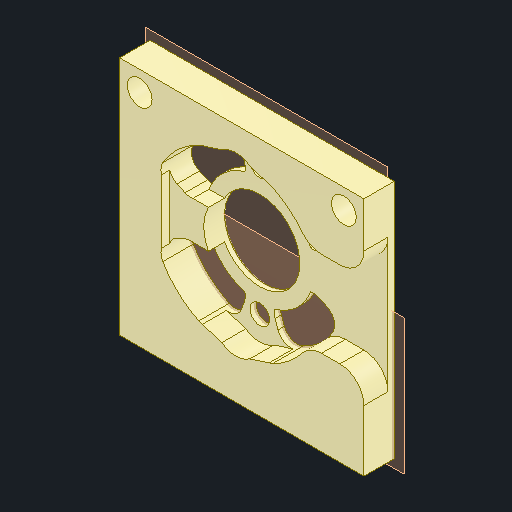
# Autodesk Inventor part: front_motur_holder
Saved by Autodesk Inventor 2023 (Build 270158000, 158)
## iProperties
Created: 2024-04-30
Part Number: front_motur_holder
Material: Nylon 6/6
Document SubType Name: Modeling
Designer: szymo
Density: 1.13 g/cm^3
Appearance: Nylon 6
Mass: 2.32105 g
Surface Area: 21.928 cm^2
Volume: 2.05403 cm^3
Author: szymo
Autodesk Inventor part; units mm, degrees
ref_plane "YZ Plane" through (0, 0, 0) normal (1, 0, 0) x (0, 1, 0)
ref_plane "XZ Plane" through (0, 0, 0) normal (0, 1, 0) x (-1, 0, 0)
ref_plane "XY Plane" through (0, 0, 0) normal (0, 0, 1) x (1, 0, 0)
ref_plane "Work Plane1" through (0, 0, 0) normal (0, 0, 1) x (1, 0, 0)
ref_plane "Work Plane2" through (-0.625, 8.3125, -0.3) normal (0, 0, 1) x (0, 1, 0)
sketch "Sketch6" plane through (-0.625, 8.3125, -0.3) normal (0, 0, 1) x (0, 1, 0)
  line L0 (-3.58, 8.0542) -> (-3.1299, 7.0416) projected
  arc A0 (-3.5233, 5.7815) -> (-3.1299, 7.0416) centre (-4.0437, 6.6354) ccw projected
  arc A1 (-3.5233, 5.7815) -> (-6.0426, 3.0539) centre (0, 0) ccw projected
  arc A2 (-7.2676, 2.5618) -> (-6.0426, 3.0539) centre (-6.9351, 3.5049) ccw projected
  line L1 (-7.2676, 2.5618) -> (-8.3126, 2.9302) projected
  arc A3 (-8.8798, 4.3099) -> (-8.3126, 2.9302) centre (-7.9802, 3.8733) ccw projected
  arc A4 (-5.0004, 8.5102) -> (-8.8798, 4.3099) centre (0, 0) ccw projected
  arc A5 (-3.58, 8.0542) -> (-5.0004, 8.5102) centre (-4.4938, 7.648) ccw projected
  line L2 (-3.1299, -7.0416) -> (-3.58, -8.0542) projected
  arc A6 (-5.0004, -8.5102) -> (-3.58, -8.0542) centre (-4.4938, -7.648) ccw projected
  arc A7 (-8.8798, -4.3099) -> (-5.0004, -8.5102) centre (0, 0) ccw projected
  arc A8 (-8.3126, -2.9302) -> (-8.8798, -4.3099) centre (-7.9802, -3.8733) ccw projected
  line L3 (-8.3126, -2.9302) -> (-7.2676, -2.5618) projected
  arc A9 (-6.0426, -3.0539) -> (-7.2676, -2.5618) centre (-6.9351, -3.5049) ccw projected
  arc A10 (-6.0426, -3.0539) -> (-3.5233, -5.7815) centre (0, 0) ccw projected
  arc A11 (-3.1299, -7.0416) -> (-3.5233, -5.7815) centre (-4.0437, -6.6354) ccw projected
  line L4 (3.1299, 7.0416) -> (3.58, 8.0542) projected
  arc A12 (5.0004, 8.5102) -> (3.58, 8.0542) centre (4.4938, 7.648) ccw projected
  arc A13 (8.8798, 4.3099) -> (5.0004, 8.5102) centre (0, 0) ccw projected
  arc A14 (8.3126, 2.9302) -> (8.8798, 4.3099) centre (7.9802, 3.8733) ccw projected
  line L5 (8.3126, 2.9302) -> (7.2676, 2.5618) projected
  arc A15 (6.0426, 3.0539) -> (7.2676, 2.5618) centre (6.9351, 3.5049) ccw projected
  arc A16 (6.0426, 3.0539) -> (3.5233, 5.7815) centre (0, 0) ccw projected
  arc A17 (3.1299, 7.0416) -> (3.5233, 5.7815) centre (4.0437, 6.6354) ccw projected
  line L6 (3.58, -8.0542) -> (3.1299, -7.0416) projected
  arc A18 (3.5233, -5.7815) -> (3.1299, -7.0416) centre (4.0437, -6.6354) ccw projected
  arc A19 (3.5233, -5.7815) -> (6.0426, -3.0539) centre (0, 0) ccw projected
  arc A20 (7.2676, -2.5618) -> (6.0426, -3.0539) centre (6.9351, -3.5049) ccw projected
  line L7 (7.2676, -2.5618) -> (8.3126, -2.9302) projected
  arc A21 (8.8798, -4.3099) -> (8.3126, -2.9302) centre (7.9802, -3.8733) ccw projected
  arc A22 (5.0004, -8.5102) -> (8.8798, -4.3099) centre (0, 0) ccw projected
  arc A23 (3.58, -8.0542) -> (5.0004, -8.5102) centre (4.4938, -7.648) ccw projected
  circle A24 centre (8, 0) radius 1.2295 projected
  circle A25 centre (-8, 0) radius 1.2295 projected
  circle A26 centre (0, 0) radius 5 projected
  circle A27 centre (0, 0) radius 13.75 projected
  line L8 (-10, 15.75) -> (14, 15.75) projected
  line L9 (-10, 15.75) -> (-10, 9.4373) projected
  arc A28 (-10, 9.4373) -> (-0.3764, -13.7448) centre (0, 0) ccw projected
  line L10 (-0.3764, -13.7448) -> (-1, -16) projected
  line L11 (14, -16) -> (-1, -16) projected
  line L12 (14, 15.75) -> (14, -16) projected
  line L13 (14, -16) -> (-16, -16)
  line L14 (-16, -16) -> (-16, 14.5)
  line L15 (-16, 14.5) -> (14, 14.5)
  line L16 (14, 14.5) -> (14, -16)
  line L17 (-19.5, 96) -> (-19.5, -16) projected
  line L18 (-19.5, -16) -> (-16, -16) projected
  line L19 (-16, 96) -> (-16, -16) projected
  line L20 (-19.5, 96) -> (-16, 96) projected
  arc A29 (3.1299, 7.0416) -> (3.5233, 5.7815) centre (4.0437, 6.6354) ccw projected
  arc A30 (6.0426, 3.0539) -> (3.5233, 5.7815) centre (0, 0) ccw projected
  arc A31 (6.0426, 3.0539) -> (7.2676, 2.5618) centre (6.9351, 3.5049) ccw projected
  line L21 (8.3126, 2.9302) -> (7.2676, 2.5618) projected
  arc A32 (8.3126, 2.9302) -> (8.8798, 4.3099) centre (7.9802, 3.8733) ccw projected
  arc A33 (8.8798, 4.3099) -> (5.0004, 8.5102) centre (0, 0) ccw projected
  arc A34 (5.0004, 8.5102) -> (3.58, 8.0542) centre (4.4938, 7.648) ccw projected
  line L22 (3.1299, 7.0416) -> (3.58, 8.0542) projected
  arc A35 (8.8798, -4.3099) -> (8.3126, -2.9302) centre (7.9802, -3.8733) ccw projected
  line L23 (7.2676, -2.5618) -> (8.3126, -2.9302) projected
  arc A36 (7.2676, -2.5618) -> (6.0426, -3.0539) centre (6.9351, -3.5049) ccw projected
  arc A37 (3.5233, -5.7815) -> (6.0426, -3.0539) centre (0, 0) ccw projected
  arc A38 (3.5233, -5.7815) -> (3.1299, -7.0416) centre (4.0437, -6.6354) ccw projected
  line L24 (3.58, -8.0542) -> (3.1299, -7.0416) projected
  arc A39 (3.58, -8.0542) -> (5.0004, -8.5102) centre (4.4938, -7.648) ccw projected
  arc A40 (5.0004, -8.5102) -> (8.8798, -4.3099) centre (0, 0) ccw projected
  arc A41 (-3.1299, -7.0416) -> (-3.5233, -5.7815) centre (-4.0437, -6.6354) ccw projected
  arc A42 (-6.0426, -3.0539) -> (-3.5233, -5.7815) centre (0, 0) ccw projected
  arc A43 (-6.0426, -3.0539) -> (-7.2676, -2.5618) centre (-6.9351, -3.5049) ccw projected
  line L25 (-8.3126, -2.9302) -> (-7.2676, -2.5618) projected
  arc A44 (-8.3126, -2.9302) -> (-8.8798, -4.3099) centre (-7.9802, -3.8733) ccw projected
  arc A45 (-8.8798, -4.3099) -> (-5.0004, -8.5102) centre (0, 0) ccw projected
  arc A46 (-5.0004, -8.5102) -> (-3.58, -8.0542) centre (-4.4938, -7.648) ccw projected
  line L26 (-3.1299, -7.0416) -> (-3.58, -8.0542) projected
  arc A47 (-3.5233, 5.7815) -> (-3.1299, 7.0416) centre (-4.0437, 6.6354) ccw projected
  line L27 (-3.58, 8.0542) -> (-3.1299, 7.0416) projected
  arc A48 (-3.58, 8.0542) -> (-5.0004, 8.5102) centre (-4.4938, 7.648) ccw projected
  arc A49 (-5.0004, 8.5102) -> (-8.8798, 4.3099) centre (0, 0) ccw projected
  arc A50 (-8.8798, 4.3099) -> (-8.3126, 2.9302) centre (-7.9802, 3.8733) ccw projected
  line L28 (-7.2676, 2.5618) -> (-8.3126, 2.9302) projected
  arc A51 (-7.2676, 2.5618) -> (-6.0426, 3.0539) centre (-6.9351, 3.5049) ccw projected
  arc A52 (-3.5233, 5.7815) -> (-6.0426, 3.0539) centre (0, 0) ccw projected
  circle A53 centre (0, 0) radius 6.7705
  arc A54 (2.4903, 7.3259) -> (2.3692, 6.3425) centre (4.0437, 6.6354) ccw
  line L29 (2.4903, 7.3259) -> (2.9403, 8.3385)
  arc A55 (5.355, 9.1137) -> (2.9403, 8.3385) centre (4.4938, 7.648) ccw
  arc A56 (9.5096, 4.6156) -> (5.355, 9.1137) centre (0, 0) ccw
  arc A57 (8.5453, 2.27) -> (9.5096, 4.6156) centre (7.9802, 3.8733) ccw
  line L30 (8.5453, 2.27) -> (7.5003, 1.9016)
  arc A58 (6.5103, 1.8588) -> (7.5003, 1.9016) centre (6.9351, 3.5049) ccw
  arc A59 (7.5003, -1.9016) -> (6.5103, -1.8588) centre (6.9351, -3.5049) ccw
  line L31 (7.5003, -1.9016) -> (8.5453, -2.27)
  arc A60 (9.5096, -4.6156) -> (8.5453, -2.27) centre (7.9802, -3.8733) ccw
  arc A61 (5.355, -9.1137) -> (9.5096, -4.6156) centre (0, 0) ccw
  arc A62 (2.9403, -8.3385) -> (5.355, -9.1137) centre (4.4938, -7.648) ccw
  line L32 (2.9403, -8.3385) -> (2.4903, -7.3259)
  arc A63 (2.3692, -6.3425) -> (2.4903, -7.3259) centre (4.0437, -6.6354) ccw
  arc A64 (-2.4903, -7.3259) -> (-2.3692, -6.3425) centre (-4.0437, -6.6354) ccw
  line L33 (-2.4903, -7.3259) -> (-2.9403, -8.3385)
  arc A65 (-5.355, -9.1137) -> (-2.9403, -8.3385) centre (-4.4938, -7.648) ccw
  arc A66 (-9.5096, -4.6156) -> (-5.355, -9.1137) centre (0, 0) ccw
  arc A67 (-8.5453, -2.27) -> (-9.5096, -4.6156) centre (-7.9802, -3.8733) ccw
  line L34 (-8.5453, -2.27) -> (-7.5003, -1.9016)
  arc A68 (-6.5103, -1.8588) -> (-7.5003, -1.9016) centre (-6.9351, -3.5049) ccw
  arc A69 (-7.5003, 1.9016) -> (-6.5103, 1.8588) centre (-6.9351, 3.5049) ccw
  line L35 (-7.5003, 1.9016) -> (-8.5453, 2.27)
  arc A70 (-9.5096, 4.6156) -> (-8.5453, 2.27) centre (-7.9802, 3.8733) ccw
  arc A71 (-5.355, 9.1137) -> (-9.5096, 4.6156) centre (0, 0) ccw
  arc A72 (-2.9403, 8.3385) -> (-5.355, 9.1137) centre (-4.4938, 7.648) ccw
  line L36 (-2.9403, 8.3385) -> (-2.4903, 7.3259)
  arc A73 (-2.3692, 6.3425) -> (-2.4903, 7.3259) centre (-4.0437, 6.6354) ccw
  point P0 (-8.3125, -0.625)
  point P1 (2.4903, 7.3259)
  point P2 (2.9403, 8.3385)
  point P3 (9.5096, 4.6156)
  point P4 (8.5453, 2.27)
  point P5 (7.5003, 1.9016)
  point P6 (3.5233, 5.7815)
  point P7 (-3.5233, 5.7815)
  point P8 (-6.0426, 3.0539)
  point P9 (-8.5453, 2.27)
  point P10 (-5.355, 9.1137)
  point P11 (-2.4903, 7.3259)
  point P12 (-3.5233, -5.7815)
  point P13 (-2.4903, -7.3259)
  point P14 (-2.9403, -8.3385)
  point P15 (-8.5453, -2.27)
  point P16 (3.5233, -5.7815)
  point P17 (6.0426, -3.0539)
  point P18 (7.5003, -1.9016)
  point P19 (8.5453, -2.27)
  point P20 (9.5096, -4.6156)
  point P21 (5.355, -9.1137)
  point P22 (2.9403, -8.3385)
  point P23 (2.4903, -7.3259)
  point P24 (14, 14.5)
  dimension "d39" = 16
  dimension "d40" = 14.5
  dimension "d41" = 0.7
  dimension "d42" = 0.7
  dimension "d43" = 0.7
  dimension "d44" = 0.7
  dimension "d45" = 0.7
  dimension "d46" = 0.7
  dimension "d47" = 0.7
  dimension "d48" = 0.7
  dimension "d49" = 0.7
  dimension "d50" = 0.7
  dimension "d51" = 0.7
  dimension "d52" = 0.7
  dimension "d53" = 0.7
  dimension "d54" = 0.7
  dimension "d55" = 0.7
  dimension "d56" = 0.7
  dimension "d57" = 0.7
  dimension "d58" = 0.7
  dimension "d59" = 0.7
  dimension "d60" = 0.7
  dimension "d61" = 0.7
  dimension "d62" = 0.7
  dimension "d63" = 0.7
  dimension "d64" = 0.7
  dimension "d65" = 0.7
  dimension "d66" = 0.7
  dimension "d67" = 0.7
  dimension "d68" = 0.7
  constraints: 40 point on circle, 24 end point, 20 centre point, 10 parallel, 1 coincident, 1 horizontal, 1 perpendicular, 1 point on line, 11 other
  measures "d39" distance from line of L11 A1.centre
  measures "d40" distance from line of L15 A1.centre
  measures "d41" radial gap between concentric circles of A17 A54
  measures "d42" distance between parallel lines of L4 L29
  measures "d43" radial gap between concentric circles of A12 A55
  measures "d44" radial gap between concentric circles of A13 A56
  measures "d45" radial gap between concentric circles of A14 A57
  measures "d46" distance between parallel lines of L5 L30
  measures "d47" radial gap between concentric circles of A15 A58
  measures "d48" radial gap between concentric circles of A20 A59
  measures "d49" distance between parallel lines of L7 L31
  measures "d50" radial gap between concentric circles of A35 A60
  measures "d51" radial gap between concentric circles of A40 A61
  measures "d52" radial gap between concentric circles of A39 A62
  measures "d53" distance between parallel lines of L6 L32
  measures "d54" radial gap between concentric circles of A18 A63
  measures "d55" radial gap between concentric circles of A11 A64
  measures "d56" distance between parallel lines of L26 L33
  measures "d57" radial gap between concentric circles of A6 A65
  measures "d58" radial gap between concentric circles of A45 A66
  measures "d59" radial gap between concentric circles of A44 A67
  measures "d60" distance between parallel lines of L3 L34
  measures "d61" radial gap between concentric circles of A9 A68
  measures "d62" radial gap between concentric circles of A2 A69
  measures "d63" distance between parallel lines of L28 L35
  measures "d64" radial gap between concentric circles of A3 A70
  measures "d65" radial gap between concentric circles of A4 A71
  measures "d66" radial gap between concentric circles of A5 A72
  measures "d67" distance between parallel lines of L27 L36
  measures "d68" radial gap between concentric circles of A47 A73
extrude "Extrusion4" add sketch "Sketch6" along normal blind 0.8 contours A53 A16 A19 A10 A1 | A27 | A27 L9 L15 L12 L11 L10 | A27 L10 L13 L14 L15 L9
sketch "Sketch7" plane through (-0.625, 8.3125, 0.5) normal (0, 0, 1) x (1, 0, 0)
  arc A0 (-7.3259, 2.4903) -> (-6.3425, 2.3692) centre (-6.6354, 4.0437) ccw projected
  line L0 (-7.3259, 2.4903) -> (-8.3385, 2.9403) projected
  arc A1 (-9.1137, 5.355) -> (-8.3385, 2.9403) centre (-7.648, 4.4938) ccw projected
  arc A2 (-4.6156, 9.5096) -> (-9.1137, 5.355) centre (0, 0) ccw projected
  arc A3 (-2.27, 8.5453) -> (-4.6156, 9.5096) centre (-3.8733, 7.9802) ccw projected
  line L1 (-2.27, 8.5453) -> (-1.9016, 7.5003) projected
  arc A4 (-1.8588, 6.5103) -> (-1.9016, 7.5003) centre (-3.5049, 6.9351) ccw projected
  arc A5 (-1.8588, 6.5103) -> (-6.3425, 2.3692) centre (0, 0) ccw projected
  arc A6 (-6.3425, -2.3692) -> (-1.8588, -6.5103) centre (0, 0) ccw projected
  arc A7 (-1.9016, -7.5003) -> (-1.8588, -6.5103) centre (-3.5049, -6.9351) ccw projected
  line L2 (-1.9016, -7.5003) -> (-2.27, -8.5453) projected
  arc A8 (-4.6156, -9.5096) -> (-2.27, -8.5453) centre (-3.8733, -7.9802) ccw projected
  arc A9 (-9.1137, -5.355) -> (-4.6156, -9.5096) centre (0, 0) ccw projected
  arc A10 (-8.3385, -2.9403) -> (-9.1137, -5.355) centre (-7.648, -4.4938) ccw projected
  line L3 (-8.3385, -2.9403) -> (-7.3259, -2.4903) projected
  arc A11 (-6.3425, -2.3692) -> (-7.3259, -2.4903) centre (-6.6354, -4.0437) ccw projected
  circle A12 centre (0, -8) radius 1.2295 projected
  arc A13 (1.8588, -6.5103) -> (6.3425, -2.3692) centre (0, 0) ccw projected
  arc A14 (7.3259, -2.4903) -> (6.3425, -2.3692) centre (6.6354, -4.0437) ccw projected
  line L4 (7.3259, -2.4903) -> (8.3385, -2.9403) projected
  arc A15 (9.1137, -5.355) -> (8.3385, -2.9403) centre (7.648, -4.4938) ccw projected
  arc A16 (4.6156, -9.5096) -> (9.1137, -5.355) centre (0, 0) ccw projected
  arc A17 (2.27, -8.5453) -> (4.6156, -9.5096) centre (3.8733, -7.9802) ccw projected
  line L5 (2.27, -8.5453) -> (1.9016, -7.5003) projected
  arc A18 (1.8588, -6.5103) -> (1.9016, -7.5003) centre (3.5049, -6.9351) ccw projected
  arc A19 (6.3425, 2.3692) -> (1.8588, 6.5103) centre (0, 0) ccw projected
  arc A20 (1.9016, 7.5003) -> (1.8588, 6.5103) centre (3.5049, 6.9351) ccw projected
  line L6 (1.9016, 7.5003) -> (2.27, 8.5453) projected
  arc A21 (4.6156, 9.5096) -> (2.27, 8.5453) centre (3.8733, 7.9802) ccw projected
  arc A22 (9.1137, 5.355) -> (4.6156, 9.5096) centre (0, 0) ccw projected
  arc A23 (8.3385, 2.9403) -> (9.1137, 5.355) centre (7.648, 4.4938) ccw projected
  line L7 (8.3385, 2.9403) -> (7.3259, 2.4903) projected
  arc A24 (6.3425, 2.3692) -> (7.3259, 2.4903) centre (6.6354, 4.0437) ccw projected
  circle A25 centre (0, 0) radius 5 projected
  circle A26 centre (0, 8) radius 1.2295 projected
  line L8 (-14.5, 14) -> (-14.5, -16) projected
  line L9 (-14.5, -16) -> (16, -16) projected
  line L10 (16, -16) -> (16, 14) projected
  line L11 (16, 14) -> (-14.5, 14) projected
  circle A27 centre (0, 8) radius 3
  circle A28 centre (0, -8) radius 1.2295 projected
  circle A29 centre (0, -8) radius 3
  arc A30 (9.1137, 5.355) -> (4.6156, 9.5096) centre (0, 0) ccw projected
  line L12 (9.1137, 5.355) -> (16, 5.355)
  line L13 (16, -16) -> (16, 14) projected
  arc A31 (9.1137, -5.355) -> (8.3385, -2.9403) centre (7.648, -4.4938) ccw projected
  line L14 (9.1137, -5.355) -> (16, -5.355)
  arc A32 (4.6156, 9.5096) -> (2.27, 8.5453) centre (3.8733, 7.9802) ccw projected
  line L15 (4.6156, 9.5096) -> (0, 11)
  arc A33 (-2.27, 8.5453) -> (-4.6156, 9.5096) centre (-3.8733, 7.9802) ccw projected
  line L16 (-4.6156, 9.5096) -> (0, 11)
  arc A34 (-9.1137, 5.355) -> (-8.3385, 2.9403) centre (-7.648, 4.4938) ccw projected
  line L17 (-9.2666, 3.9741) -> (-9.2666, -3.9741)
  arc A35 (-8.3385, -2.9403) -> (-9.1137, -5.355) centre (-7.648, -4.4938) ccw projected
  arc A36 (-4.6156, -9.5096) -> (-2.27, -8.5453) centre (-3.8733, -7.9802) ccw projected
  line L18 (-4.6156, -9.5096) -> (0, -11)
  arc A37 (2.27, -8.5453) -> (4.6156, -9.5096) centre (3.8733, -7.9802) ccw projected
  line L19 (0, -11) -> (4.6156, -9.5096)
  line L20 (-6.3425, 2.3692) -> (-4.4031, 2.3692)
  circle A38 centre (0, 0) radius 5 projected
  arc A39 (-6.3425, -2.3692) -> (-1.8588, -6.5103) centre (0, 0) ccw projected
  line L21 (-6.3425, -2.3692) -> (-4.4031, -2.3692)
  point P0 (0.625, -8.3125)
  point P1 (-4.1656, 9.6549)
  point P2 (-1.7545, 10.4334)
  point P3 (1.7545, 10.4334)
  point P4 (4.1656, 9.6549)
  point P5 (4.1656, -9.6549)
  point P6 (1.7545, -10.4334)
  point P7 (-1.7545, -10.4334)
  point P8 (-4.1656, -9.6549)
  point P9 (-2.4735, -6.3025)
  point P10 (0, -5)
  point P11 (0, 5)
  point P12 (-2.4735, 6.3025)
  dimension "d71" = 6
  dimension "d72" = 6
  constraints: 18 end point, 5 point on circle, 2 coincident, 2 horizontal, 2 parallel, 2 point on line, 10 other
extrude "Extrusion5" add sketch "Sketch7" along normal blind 2 contours A0 L20 A25 L21 A11 L3 A10 L17 A1 L0 | L17 A10 A9 A8 L18 A29 L19 A17 A16 L14 L10 L9 L8 L11 L12 A22 A21 L15 A27 L16 A3 A2 A1
fillet "Fillet1" radius 3 4 edges at (15.375, 13.6675, 1.5) (15.375, 2.9575, 1.5) (8.4887, 2.9575, 1.5) (8.4887, 13.6675, 1.5)
fillet "Fillet2" radius 0.2 1 edges at (-0.625, 3.3125, -0.3)
sketch "Sketch8" plane through (-0.625, 8.3125, -0.3) normal (0, 0, -1) x (-1, 0, 0)
  line L0 (14.5, 14) -> (14.5, -16) projected
  line L1 (-16, 14) -> (14.5, 14) projected
  line L2 (-16, -16) -> (-16, 14) projected
  line L3 (14.5, -16) -> (-16, -16) projected
  circle A0 centre (0, 8) radius 1.2295 projected
  arc A1 (-1.8588, 6.5103) -> (-6.3425, 2.3692) centre (0, 0) ccw projected
  arc A2 (-7.3259, 2.4903) -> (-6.3425, 2.3692) centre (-6.6354, 4.0437) ccw projected
  line L4 (-8.3385, 2.9403) -> (-7.3259, 2.4903) projected
  arc A3 (-9.1137, 5.355) -> (-8.3385, 2.9403) centre (-7.648, 4.4938) ccw projected
  arc A4 (-4.6156, 9.5096) -> (-9.1137, 5.355) centre (0, 0) ccw projected
  arc A5 (-2.27, 8.5453) -> (-4.6156, 9.5096) centre (-3.8733, 7.9802) ccw projected
  line L5 (-1.9016, 7.5003) -> (-2.27, 8.5453) projected
  arc A6 (-1.8588, 6.5103) -> (-1.9016, 7.5003) centre (-3.5049, 6.9351) ccw projected
  arc A7 (-6.3425, -2.3692) -> (-1.8588, -6.5103) centre (0, 0) ccw projected
  arc A8 (-1.9016, -7.5003) -> (-1.8588, -6.5103) centre (-3.5049, -6.9351) ccw projected
  line L6 (-2.27, -8.5453) -> (-1.9016, -7.5003) projected
  arc A9 (-4.6156, -9.5096) -> (-2.27, -8.5453) centre (-3.8733, -7.9802) ccw projected
  arc A10 (-9.1137, -5.355) -> (-4.6156, -9.5096) centre (0, 0) ccw projected
  arc A11 (-8.3385, -2.9403) -> (-9.1137, -5.355) centre (-7.648, -4.4938) ccw projected
  line L7 (-7.3259, -2.4903) -> (-8.3385, -2.9403) projected
  arc A12 (-6.3425, -2.3692) -> (-7.3259, -2.4903) centre (-6.6354, -4.0437) ccw projected
  circle A13 centre (0, -8) radius 1.2295 projected
  arc A14 (1.8588, -6.5103) -> (6.3425, -2.3692) centre (0, 0) ccw projected
  arc A15 (7.3259, -2.4903) -> (6.3425, -2.3692) centre (6.6354, -4.0437) ccw projected
  line L8 (8.3385, -2.9403) -> (7.3259, -2.4903) projected
  arc A16 (9.1137, -5.355) -> (8.3385, -2.9403) centre (7.648, -4.4938) ccw projected
  arc A17 (4.6156, -9.5096) -> (9.1137, -5.355) centre (0, 0) ccw projected
  arc A18 (2.27, -8.5453) -> (4.6156, -9.5096) centre (3.8733, -7.9802) ccw projected
  line L9 (1.9016, -7.5003) -> (2.27, -8.5453) projected
  arc A19 (1.8588, -6.5103) -> (1.9016, -7.5003) centre (3.5049, -6.9351) ccw projected
  arc A20 (6.3425, 2.3692) -> (7.3259, 2.4903) centre (6.6354, 4.0437) ccw projected
  arc A21 (6.3425, 2.3692) -> (1.8588, 6.5103) centre (0, 0) ccw projected
  arc A22 (1.9016, 7.5003) -> (1.8588, 6.5103) centre (3.5049, 6.9351) ccw projected
  line L10 (2.27, 8.5453) -> (1.9016, 7.5003) projected
  arc A23 (4.6156, 9.5096) -> (2.27, 8.5453) centre (3.8733, 7.9802) ccw projected
  arc A24 (9.1137, 5.355) -> (4.6156, 9.5096) centre (0, 0) ccw projected
  arc A25 (8.3385, 2.9403) -> (9.1137, 5.355) centre (7.648, 4.4938) ccw projected
  line L11 (7.3259, 2.4903) -> (8.3385, 2.9403) projected
  circle A26 centre (0, 0) radius 5.2 projected
  circle A27 centre (-13.5, 11.5) radius 2.5
  circle A28 centre (12, 11.5) radius 2.5
  point P0 (-0.625, -8.3125)
  dimension "d77" = 5
  dimension "d78" = 2.5
  dimension "d79" = 2.5
  dimension "d80" = 5
  dimension "d81" = 2.5
  dimension "d82" = 2.5
  constraints: 2 centre point, 2 coincident
  measures "d77" diameter of A27
  measures "d78" distance from line of L1 A27.centre
  measures "d79" distance from line of L2 A27.centre
  measures "d80" diameter of A28
  measures "d81" distance from line of L1 A28.centre
  measures "d82" distance from line of L0 A28.centre
hole "Hole3" at (12.875, 19.8125, -0.3) at (-12.625, 19.8125, -0.3) direction (0, 0, 1) diameter 3.1 end through all countersink diameter 5 countersink angle 90 clearance for "Countersunk Flat Head Screw ISO 2009/7046" size "M2.5" standard "ISO"
sketch "Sketch9" plane through (-0.625, 8.3125, 2.5) normal (0, 0, 1) x (1, 0, 0)
  circle A0 centre (13.5, 11.5) radius 1.55 projected
  circle A1 centre (-12, 11.5) radius 1.55 projected
  arc A2 (8.3296, 6.508) -> (10.6936, 5.355) centre (10.6936, 8.355) ccw projected
  line L0 (10.6936, 5.355) -> (13, 5.355) projected
  arc A3 (13, 5.355) -> (16, 8.355) centre (13, 8.355) ccw projected
  line L1 (16, 8.355) -> (16, 14) projected
  line L2 (16, 14) -> (-14.5, 14) projected
  line L3 (-14.5, 14) -> (-14.5, -16) projected
  line L4 (-14.5, -16) -> (16, -16) projected
  line L5 (16, -16) -> (16, -8.355) projected
  arc A4 (16, -8.355) -> (13, -5.355) centre (13, -8.355) ccw projected
  line L6 (13, -5.355) -> (10.6936, -5.355) projected
  arc A5 (10.6936, -5.355) -> (8.3296, -6.508) centre (10.6936, -8.355) ccw projected
  arc A6 (4.6156, -9.5096) -> (8.3296, -6.508) centre (0, 0) ccw projected
  arc A7 (4.1656, -9.6549) -> (4.6156, -9.5096) centre (3.8733, -7.9802) ccw projected
  line L7 (4.1656, -9.6549) -> (1.7545, -10.4334) projected
  arc A8 (-1.7545, -10.4334) -> (1.7545, -10.4334) centre (0, -8) ccw projected
  line L8 (-1.7545, -10.4334) -> (-4.1656, -9.6549) projected
  arc A9 (-4.6156, -9.5096) -> (-4.1656, -9.6549) centre (-3.8733, -7.9802) ccw projected
  arc A10 (-9.1137, -5.355) -> (-4.6156, -9.5096) centre (0, 0) ccw projected
  arc A11 (-8.3385, -2.9403) -> (-9.1137, -5.355) centre (-7.648, -4.4938) ccw projected
  line L9 (-8.3385, -2.9403) -> (-7.3259, -2.4903) projected
  arc A12 (-6.3425, -2.3692) -> (-7.3259, -2.4903) centre (-6.6354, -4.0437) ccw projected
  line L10 (-6.3425, -2.3692) -> (-4.4031, -2.3692) projected
  arc A13 (-4.4031, 2.3692) -> (-4.4031, -2.3692) centre (0, 0) ccw projected
  line L11 (-4.4031, 2.3692) -> (-6.3425, 2.3692) projected
  arc A14 (-7.3259, 2.4903) -> (-6.3425, 2.3692) centre (-6.6354, 4.0437) ccw projected
  line L12 (-7.3259, 2.4903) -> (-8.3385, 2.9403) projected
  arc A15 (-9.1137, 5.355) -> (-8.3385, 2.9403) centre (-7.648, 4.4938) ccw projected
  arc A16 (-4.6156, 9.5096) -> (-9.1137, 5.355) centre (0, 0) ccw projected
  arc A17 (-4.1656, 9.6549) -> (-4.6156, 9.5096) centre (-3.8733, 7.9802) ccw projected
  line L13 (-4.1656, 9.6549) -> (-1.7545, 10.4334) projected
  arc A18 (1.7545, 10.4334) -> (-1.7545, 10.4334) centre (0, 8) ccw projected
  line L14 (1.7545, 10.4334) -> (4.1656, 9.6549) projected
  arc A19 (4.6156, 9.5096) -> (4.1656, 9.6549) centre (3.8733, 7.9802) ccw projected
  arc A20 (8.3296, 6.508) -> (4.6156, 9.5096) centre (0, 0) ccw projected
  arc A21 (-9.1137, 5.355) -> (-8.3385, 2.9403) centre (-7.648, 4.4938) ccw projected
  line L15 (-9.2666, 3.9741) -> (-9.2666, -3.9741)
  point P0 (0.625, -8.3125)
  constraints: 3 point on circle, 2 end point
extrude "Extrusion6" add sketch "Sketch9" along normal blind 1 contours A20 A19 L14 A18 L13 A17 A16 A15 L15 A11 A10 A9 L8 A8 L7 A7 A6 A5 L6 A4 L5 L4 L3 L2 L1 A3 L0 A2
body "Solid2"
